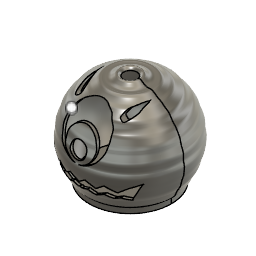
pumpkin hp (Autodesk Fusion 360 design; units mm, degrees)
Autodesk Fusion 360 part; units mm, degrees
note: some values were not read from the file. Set by a fixed rule: which sketch regions a step uses.
sketch "Sketch1" plane through (0, 0, 0) normal (0, 0, 1) x (1, 0, 0)
  line L0 (0, 15) -> (0, 0) construction
  line L1 (0, 45) -> (0, -15)
  arc A0 (0, -15) -> (0, 45) centre (0, 15) ccw
  spline S0 degree 5 poles (0, 39) (0.0615, 39.1015) (0.1845, 39.2977) (0.3695, 39.5721) (0.6169, 39.8981) (0.9276, 40.2413) (1.2404, 40.5273) (1.5563, 40.7701) (1.8774, 40.9932) (2.2063, 41.2305) (2.5456, 41.5152) (2.8972, 41.8703) (3.2609, 42.2998) (3.6342, 42.7767) (4.0126, 43.2499) (4.3918, 43.659) (4.7692, 43.9466) (5.1454, 44.0706) (5.5264, 44.019) (5.9232, 43.8147) (6.3478, 43.5011) (6.8096, 43.1332) (7.3125, 42.7664) (7.8498, 42.445) (8.4064, 42.1983) (8.9632, 42.0416) (9.5018, 41.9759) (10.0079, 41.9876) (10.4765, 42.049) (10.9152, 42.1179) (11.34, 42.1472) (11.7691, 42.0952) (12.2184, 41.9344) (12.6953, 41.6635) (13.1973, 41.3077) (13.7157, 40.9064) (14.2377, 40.5049) (14.7499, 40.1436) (15.2399, 39.8495) (15.7001, 39.6239) (16.1288, 39.4431) (16.528, 39.272) (16.9036, 39.0751) (17.2641, 38.8277) (17.6198, 38.5292) (17.981, 38.1986) (18.3569, 37.863) (18.7532, 37.5479) (19.1709, 37.2675) (19.604, 37.0133) (20.0418, 36.7611) (20.4719, 36.4798) (20.8827, 36.1412) (21.2663, 35.7275) (21.6215, 35.242) (21.9532, 34.7072) (22.2695, 34.1546) (22.5802, 33.6191) (22.8938, 33.1299) (23.2161, 32.7044) (23.5469, 32.3386) (23.8815, 32.0107) (24.2126, 31.6912) (24.5328, 31.351) (24.8366, 30.9695) (25.123, 30.5447) (25.3943, 30.0893) (25.6542, 29.6228) (25.9061, 29.165) (26.1517, 28.73) (26.3883, 28.318) (26.6101, 27.9164) (26.8105, 27.5072) (26.9844, 27.0732) (27.1306, 26.6039) (27.2537, 26.102) (27.3634, 25.5806) (27.4709, 25.0574) (27.5873, 24.5502) (27.7211, 24.0725) (27.8758, 23.6275) (28.0492, 23.209) (28.2354, 22.805) (28.4247, 22.4006) (28.6056, 21.9814) (28.7648, 21.5364) (28.8902, 21.0586) (28.973, 20.5457) (29.0102, 20.0002) (29.007, 19.4306) (28.9794, 18.8513) (28.9485, 18.2797) (28.9365, 17.7322) (28.961, 17.221) (29.0311, 16.7511) (29.1402, 16.3155) (29.2684, 15.897) (29.3902, 15.4745) (29.4815, 15.0291) (29.5266, 14.5499) (29.5257, 14.0398) (29.49, 13.5111) (29.4353, 12.9801) (29.3772, 12.4621) (29.3253, 11.9667) (29.2769, 11.4916) (29.2203, 11.0258) (29.1408, 10.5547) (29.026, 10.065) (28.8704, 9.5488) (28.6819, 9.0094) (28.4774, 8.4577) (28.2773, 7.9082) (28.1004, 7.3752) (27.9592, 6.8693) (27.8539, 6.3925) (27.7698, 5.9364) (27.6845, 5.4877) (27.5741, 5.032) (27.4185, 4.5581) (27.2095, 4.0637) (26.9519, 3.5557) (26.6595, 3.0462) (26.351, 2.5488) (26.0466, 2.075) (25.7645, 1.6301) (25.5165, 1.2097) (25.3073, 0.8024) (25.1346, 0.3947) (24.9886, -0.0239) (24.8515, -0.457) (24.6979, -0.8964) (24.5012, -1.3288) (24.2404, -1.7401) (23.9062, -2.1218) (23.5086, -2.4762) (23.0792, -2.8193) (22.6583, -3.1722) (22.2851, -3.5549) (21.9869, -3.9791) (21.7689, -4.4419) (21.6034, -4.9183) (21.4435, -5.3724) (21.2396, -5.7685) (20.9525, -6.0822) (20.5711, -6.3123) (20.1209, -6.488) (19.6468, -6.6526) (19.1978, -6.8503) (18.8132, -7.1132) (18.5044, -7.4448) (18.2519, -7.8187) (18.0219, -8.1964) (17.7767, -8.5392) (17.4886, -8.8235) (17.1512, -9.0539) (16.7732, -9.253) (16.3699, -9.4506) (15.9569, -9.6735) (15.5411, -9.933) (15.121, -10.2257) (14.6907, -10.5386) (14.2422, -10.8533) (13.7684, -11.1505) (13.2668, -11.415) (12.7398, -11.6369) (12.1934, -11.8108) (11.6358, -11.9341) (11.0757, -12.0065) (10.5216, -12.0285) (9.9799, -12.0006) (9.4549, -11.9242) (8.9485, -11.8034) (8.4604, -11.6463) (7.9881, -11.4666) (7.5262, -11.2856) (7.0678, -11.1297) (6.6058, -11.0232) (6.1347, -10.9824) (5.6519, -11.0106) (5.1595, -11.0897) (4.6635, -11.1863) (4.1714, -11.2616) (3.691, -11.2804) (3.2281, -11.2201) (2.7846, -11.0814) (2.3591, -10.8837) (1.9482, -10.6569) (1.5479, -10.4339) (1.1545, -10.2427) (0.7658, -10.0995) (0.4578, -10.0301) (0.2283, -10.0047) (0.076, -9.9996) (0, -10) knots 0 0 0 0 0 0 0.00526316 0.01052632 0.01578947 0.02105263 0.02631579 0.03157895 0.03684211 0.04210526 0.04736842 0.05263158 0.05789474 0.06315789 0.06842105 0.07368421 0.07894737 0.08421053 0.08947368 0.09473684 0.1 0.10526316 0.11052632 0.11578947 0.12105263 0.12631579 0.13157895 0.13684211 0.14210526 0.14736842 0.15263158 0.15789474 0.16315789 0.16842105 0.17368421 0.17894737 0.18421053 0.18947368 0.19473684 0.2 0.20526316 0.21052632 0.21578947 0.22105263 0.22631579 0.23157895 0.23684211 0.24210526 0.24736842 0.25263158 0.25789474 0.26315789 0.26842105 0.27368421 0.27894737 0.28421053 0.28947368 0.29473684 0.3 0.30526316 0.31052632 0.31578947 0.32105263 0.32631579 0.33157895 0.33684211 0.34210526 0.34736842 0.35263158 0.35789474 0.36315789 0.36842105 0.37368421 0.37894737 0.38421053 0.38947368 0.39473684 0.4 0.40526316 0.41052632 0.41578947 0.42105263 0.42631579 0.43157895 0.43684211 0.44210526 0.44736842 0.45263158 0.45789474 0.46315789 0.46842105 0.47368421 0.47894737 0.48421053 0.48947368 0.49473684 0.5 0.50526316 0.51052632 0.51578947 0.52105263 0.52631579 0.53157895 0.53684211 0.54210526 0.54736842 0.55263158 0.55789474 0.56315789 0.56842105 0.57368421 0.57894737 0.58421053 0.58947368 0.59473684 0.6 0.60526316 0.61052632 0.61578947 0.62105263 0.62631579 0.63157895 0.63684211 0.64210526 0.64736842 0.65263158 0.65789474 0.66315789 0.66842105 0.67368421 0.67894737 0.68421053 0.68947368 0.69473684 0.7 0.70526316 0.71052632 0.71578947 0.72105263 0.72631579 0.73157895 0.73684211 0.74210526 0.74736842 0.75263158 0.75789474 0.76315789 0.76842105 0.77368421 0.77894737 0.78421053 0.78947368 0.79473684 0.8 0.80526316 0.81052632 0.81578947 0.82105263 0.82631579 0.83157895 0.83684211 0.84210526 0.84736842 0.85263158 0.85789474 0.86315789 0.86842105 0.87368421 0.87894737 0.88421053 0.88947368 0.89473684 0.9 0.90526316 0.91052632 0.91578947 0.92105263 0.92631579 0.93157895 0.93684211 0.94210526 0.94736842 0.95263158 0.95789474 0.96315789 0.96842105 0.97368421 0.97894737 0.98421053 0.98947368 0.99473684 1 1 1 1 1 1
  point P0 (1.4927, 40.7168)
  point P1 (3, 42)
  point P2 (5, 44)
  point P3 (7, 43)
  point P4 (10, 42)
  point P5 (12, 42)
  point P6 (15, 40)
  point P7 (17, 39)
  point P8 (18.8164, 37.5146)
  point P9 (21, 36)
  point P10 (23, 33)
  point P11 (24.5909, 31.2675)
  point P12 (26, 29)
  point P13 (27, 27)
  point P14 (27.6357, 24.3905)
  point P15 (28.4231, 22.3957)
  point P16 (29, 20)
  point P17 (29, 17)
  point P18 (29.473, 15)
  point P19 (29.3681, 12.369)
  point P20 (29, 10)
  point P21 (28, 7)
  point P22 (27.4782, 4.757)
  point P23 (26, 2)
  point P24 (25, 0)
  point P25 (24, -2)
  point P26 (22, -4)
  point P27 (21, -6)
  point P28 (19, -7)
  point P29 (17.7664, -8.5244)
  point P30 (16.2441, -9.5219)
  point P31 (14, -11)
  point P32 (11, -12)
  point P33 (8.2647, -11.5692)
  point P34 (6, -11)
  point P35 (3.5925, -11.2542)
  point P36 (1.5977, -10.4668)
  dimension "d1" = 15
  constraint coincident L0.start A0.centre
  constraint coincident L0.end origin
  constraint vertical L0
  constraint vertical L1
  constraint coincident L1 S0.end
  measures "d1" distance of L0.start L0.end
revolve "Revolve1" add sketch "Sketch1" angle 360 about axis through (0, 45, 0) along (0, -1, 0) makes body 1 in component "Pumpkin HP"
shell "Shell1" thickness 2 removed faces 0 bodies 1 in component "Pumpkin HP"
revolve "Revolve2" cut sketch "Sketch1" angle 360 about axis through (0, 45, 0) along (0, -1, 0) contours L1 A0 S0 bodies 1 in component "Pumpkin HP"
sketch "Sketch1 (2)" plane through (0, 0, 0) normal (0, 1, 0) x (1, 0, 0) in component "Pumpkin HP"
  line L0 (-37.1378, 34.2144) -> (33.8896, 34.2144)
  line L1 (33.8896, 34.2144) -> (33.8896, -30.9662)
  line L2 (33.8896, -30.9662) -> (-37.1378, -30.9662)
  line L3 (-37.1378, -30.9662) -> (-37.1378, 34.2144)
  constraint horizontal L0
  constraint vertical L1
  constraint horizontal L2
  constraint vertical L3
extrude "Extrude1" cut sketch "Sketch1 (2)" against normal blind 25 from surface at -3.5 bodies 1 in component "Pumpkin HP"
ref_plane "WorkPlane1" through (0, 0, 32) normal (0, 0, 1) x (1, 0, 0) in component "Pumpkin HP"
sketch "Sketch2" plane through (0, 0, 32) normal (0, 0, 1) x (1, 0, 0) in component "Pumpkin HP"
  line L0 (0, 43) -> (0, 44)
sketch "Sketch3" plane through (0, 0, 0) normal (0, 0, 1) x (1, 0, 0) in component "Pumpkin HP"
sketch "Sketch2 (2)" plane through (0, 0, 0) normal (0, 0, 1) x (1, 0, 0)
  circle A0 centre (0, 28) radius 12.0416
  circle A1 centre (0, 24) radius 8.0623
  circle A2 centre (0, 22) radius 4.2846
  line L0 (0, 7) -> (-4, 10)
  line L1 (-4, 10) -> (-8, 7)
  line L2 (-8, 7) -> (-12, 10)
  line L3 (-12, 10) -> (-16, 7)
  line L4 (-16, 7) -> (-20, 10)
  line L5 (-20, 10) -> (-24, 12)
  line L6 (-24, 12) -> (-19.4, 2.8)
  line L7 (-19.4, 2.8) -> (-16.4069, 4.2965)
  line L8 (-16.4069, 4.2965) -> (-14.1356, 3.4322)
  line L9 (-14.1356, 3.4322) -> (-11, 5)
  line L10 (-11, 5) -> (-7, 3)
  line L11 (-7, 3) -> (-4, 5)
  line L12 (-4, 5) -> (-0.8415, 3.798)
  line L13 (-0.8415, 3.798) -> (0, 4.4619)
  spline S0 degree 5 poles (-14.3556, 40.0667) (-14.4061, 40.0411) (-14.5028, 39.9805) (-14.6337, 39.862) (-14.7796, 39.6543) (-14.9176, 39.3376) (-15.0173, 38.9957) (-15.0854, 38.6595) (-15.1266, 38.3535) (-15.1413, 38.0878) (-15.1243, 37.8543) (-15.0678, 37.6348) (-14.9643, 37.4081) (-14.8098, 37.1569) (-14.6072, 36.8763) (-14.3673, 36.5777) (-14.1054, 36.2826) (-13.8385, 36.0175) (-13.5815, 35.809) (-13.3442, 35.6781) (-13.1286, 35.6354) (-12.9248, 35.6757) (-12.7176, 35.783) (-12.4921, 35.9361) (-12.2387, 36.1126) (-11.96, 36.2951) (-11.6733, 36.4738) (-11.4025, 36.6445) (-11.1733, 36.8077) (-11.0066, 36.967) (-10.9134, 37.1279) (-10.8874, 37.2965) (-10.9098, 37.478) (-10.9579, 37.6757) (-11.0114, 37.8894) (-11.0607, 38.1138) (-11.105, 38.3402) (-11.1488, 38.5583) (-11.1995, 38.7583) (-11.2639, 38.9324) (-11.3465, 39.0766) (-11.4512, 39.1914) (-11.5815, 39.282) (-11.7422, 39.3595) (-11.9384, 39.4392) (-12.1737, 39.5347) (-12.4487, 39.6545) (-12.7592, 39.7968) (-13.0942, 39.9457) (-13.439, 40.0762) (-13.7766, 40.16) (-14.0278, 40.1687) (-14.1993, 40.1343) (-14.305, 40.0923) (-14.3556, 40.0667) knots 0 0 0 0 0 0 0.02 0.04 0.06 0.08 0.1 0.12 0.14 0.16 0.18 0.2 0.22 0.24 0.26 0.28 0.3 0.32 0.34 0.36 0.38 0.4 0.42 0.44 0.46 0.48 0.5 0.52 0.54 0.56 0.58 0.6 0.62 0.64 0.66 0.68 0.7 0.72 0.74 0.76 0.78 0.8 0.82 0.84 0.86 0.88 0.9 0.92 0.94 0.96 0.98 1 1 1 1 1 1
  line L14 (0, 43) -> (0, -4)
  spline S1 degree 5 poles (14.3556, 40.0667) (14.4061, 40.0411) (14.5028, 39.9805) (14.6337, 39.862) (14.7796, 39.6543) (14.9176, 39.3376) (15.0173, 38.9957) (15.0854, 38.6595) (15.1266, 38.3535) (15.1413, 38.0878) (15.1243, 37.8543) (15.0678, 37.6348) (14.9643, 37.4081) (14.8098, 37.1569) (14.6072, 36.8763) (14.3673, 36.5777) (14.1054, 36.2826) (13.8385, 36.0175) (13.5815, 35.809) (13.3442, 35.6781) (13.1286, 35.6354) (12.9248, 35.6757) (12.7176, 35.783) (12.4921, 35.9361) (12.2387, 36.1126) (11.96, 36.2951) (11.6733, 36.4738) (11.4025, 36.6445) (11.1733, 36.8077) (11.0066, 36.967) (10.9134, 37.1279) (10.8874, 37.2965) (10.9098, 37.478) (10.9579, 37.6757) (11.0114, 37.8894) (11.0607, 38.1138) (11.105, 38.3402) (11.1488, 38.5583) (11.1995, 38.7583) (11.2639, 38.9324) (11.3465, 39.0766) (11.4512, 39.1914) (11.5815, 39.282) (11.7422, 39.3595) (11.9384, 39.4392) (12.1737, 39.5347) (12.4487, 39.6545) (12.7592, 39.7968) (13.0942, 39.9457) (13.439, 40.0762) (13.7766, 40.16) (14.0278, 40.1687) (14.1993, 40.1343) (14.305, 40.0923) (14.3556, 40.0667) knots 0 0 0 0 0 0 0.02 0.04 0.06 0.08 0.1 0.12 0.14 0.16 0.18 0.2 0.22 0.24 0.26 0.28 0.3 0.32 0.34 0.36 0.38 0.4 0.42 0.44 0.46 0.48 0.5 0.52 0.54 0.56 0.58 0.6 0.62 0.64 0.66 0.68 0.7 0.72 0.74 0.76 0.78 0.8 0.82 0.84 0.86 0.88 0.9 0.92 0.94 0.96 0.98 1 1 1 1 1 1
  line L15 (-13.7197, 40.3889) -> (-14.9914, 39.7445)
  line L16 (13.7197, 40.3889) -> (14.9914, 39.7445)
  circle A3 centre (0, 28) radius 12.0416
  circle A4 centre (0, 24) radius 8.0623
  line L17 (0, 7) -> (4, 10)
  line L18 (4, 10) -> (8, 7)
  line L19 (8, 7) -> (12, 10)
  line L20 (12, 10) -> (16, 7)
  line L21 (16, 7) -> (20, 10)
  line L22 (20, 10) -> (24, 12)
  line L23 (24, 12) -> (19.4, 2.8)
  line L24 (19.4, 2.8) -> (16.4069, 4.2965)
  line L25 (16.4069, 4.2965) -> (14.1356, 3.4322)
  line L26 (14.1356, 3.4322) -> (11, 5)
  line L27 (11, 5) -> (7, 3)
  line L28 (7, 3) -> (4, 5)
  line L29 (4, 5) -> (0.8415, 3.798)
  line L30 (0.8415, 3.798) -> (0, 4.4619)
  point P0 (-15.1148, 38.4127)
  point P1 (-14.8436, 37.2196)
  point P2 (-13.3523, 35.7011)
  point P3 (-12.3219, 36.0536)
  point P4 (-11, 37)
  point P5 (-10.9661, 37.7077)
  point P6 (-11.183, 38.6838)
  point P7 (-11.5084, 39.2261)
  point P8 (-12.4575, 39.66)
  point P9 (15.1148, 38.4127)
  point P10 (14.8436, 37.2196)
  point P11 (13.3523, 35.7011)
  point P12 (12.3219, 36.0536)
  point P13 (11, 37)
  point P14 (10.9661, 37.7077)
  point P15 (11.183, 38.6838)
  point P16 (11.5084, 39.2261)
  point P17 (12.4575, 39.66)
  constraint parallel L0 L2
  constraint parallel L1 L3
  constraint parallel L2 L4
  constraint perpendicular L6 L7
  constraint perpendicular L6 L9
  constraint parallel L8 L12
  constraint midpoint S0.start L15
  constraint symmetric A0 L14 A3
  constraint symmetric A1 L14 A4
  constraint symmetric L0.start L14 L17.start
  constraint symmetric L0.end L14 L17.end
  constraint symmetric L1.end L14 L18.end
  constraint symmetric L2.end L14 L19.end
  constraint symmetric L3.end L14 L20.end
  constraint symmetric L4.end L14 L21.end
  constraint symmetric L5.end L14 L22.end
  constraint symmetric L6.end L14 L23.end
  constraint symmetric L7.end L14 L24.end
  constraint symmetric L8.end L14 L25.end
  constraint symmetric L9.end L14 L26.end
  constraint symmetric L10.end L14 L27.end
  constraint symmetric L11.end L14 L28.end
  constraint symmetric L12.end L14 L29.end
  constraint symmetric L13.end L14 L30.end
  constraint symmetric S0.start L14 S1.start
  constraint symmetric P0 L14 P9
  constraint symmetric P1 L14 P10
  constraint symmetric P2 L14 P11
  constraint symmetric P3 L14 P12
  constraint symmetric P4 L14 P13
  constraint symmetric P5 L14 P14
  constraint symmetric P6 L14 P15
  constraint symmetric P7 L14 P16
  constraint symmetric P8 L14 P17
  constraint symmetric L14 L15.start L16.start
  constraint symmetric L14 L15.end L16.end
sketch "Sketch3 (2)" plane through (0, 0, 0) normal (0, 0, 1) x (1, 0, 0)
sketch "Sketch4" plane through (0, 0, 0) normal (0, 0, 1) x (1, 0, 0)
sketch "Sketch5" plane through (0, 0, 0) normal (0, 0, 1) x (1, 0, 0)
extrude "Extrude2" cut sketch "Sketch2 (2)" along normal blind 100 contours A0 A1 L14 A3 A4 | A0 A1 L14 A3 A4 | A2 L14 | A2 L14 | L0 L1 L2 L3 L4 L5 L6 L7 L8 L9 L10 L11 L12 L13 L14 | L14 L17 L18 L19 L20 L21 L22 L23 L24 L25 L26 L27 L28 L29 L30 | S0 | S1 picked at (0.5712, 37.341) picked at (-0.5825, 37.3393) bodies 1 in component "Pumpkin HP"
sketch "Sketch1 (3)" plane through (0, -3.5, 0) normal (0, -1, 0) x (1, 0, 0) in component "LED Candle Lid"
  spline S0 degree 3 poles (22.359, 0) (22.359, -0.1659) (22.3571, -0.3318) (22.2886, -3.4086) (21.6558, -6.2788) (20.4908, -8.9471) (19.8312, -10.4578) (19.0065, -11.8909) (17.0571, -14.5498) (15.9384, -15.7673) (12.5018, -18.7644) (9.9548, -20.2312) (4.4419, -22.1059) (1.5287, -22.4958) (-4.2832, -22.1372) (-7.1263, -21.3919) (-12.3669, -18.8536) (-14.7142, -17.0848) (-18.5988, -12.747) (-20.0988, -10.2194) (-22.0457, -4.7316) (-22.4738, -1.8237) (-22.1915, 3.9923) (-21.4836, 6.845) (-19.0143, 12.1184) (-17.2764, 14.4888) (-12.9899, 18.4299) (-10.4823, 19.963) (-5.0205, 21.9817) (-2.1185, 22.448) (3.7008, 22.2419) (6.5625, 21.5716) (11.8679, 19.1717) (14.2608, 17.4651) (18.2579, 13.2307) (19.8237, 10.7433) (21.8543, 5.4635) (22.359, 2.7426) (22.359, 0) knots -0.923255 -0.923255 -0.923255 -0.923255 -0.87344 -0.87344 0 0 0 0.494534 0.494534 0.989069 0.989069 1.862509 1.862509 2.735949 2.735949 3.609389 3.609389 4.482829 4.482829 5.35627 5.35627 6.22971 6.22971 7.10315 7.10315 7.97659 7.97659 8.85003 8.85003 9.72347 9.72347 10.596911 10.596911 11.470351 11.470351 12.343791 12.343791 13.167416 13.167416 13.167416 13.167416
  circle A0 centre (0, 0) radius 21.0178
  circle A1 centre (0, 0) radius 20.7178
  circle A2 centre (0, 0) radius 19.25
  circle A3 centre (0, 0) radius 20.25
  dimension "d11" = -0.3
  dimension "d12" = 38.5
  dimension "d13" = 40.5
  constraint concentric A0 A2
  constraint concentric A0 A3
  measures "d12" diameter of A2
  measures "d13" diameter of A3
extrude "Extrude1'" add sketch "Sketch1 (3)" along normal blind 3 separate body contours S0 | A0 | A1 | A2 | A3 makes body 2 in component "LED Candle Lid"
component "Pumpkin HP" placed x (1, 0, 0) y (0, 1, 0) z (0, 0, 1) at (0, 0, 0)
component "LED Candle Lid" placed x (1, 0, 0) y (0, 1, 0) z (0, 0, 1) at (0, 0, 0)
